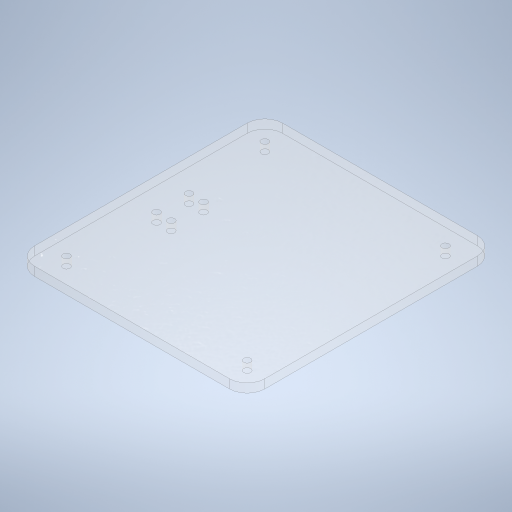
# Autodesk Inventor part: base
Saved by Autodesk Inventor 2023.1 (Build 271208000, 208)
## iProperties
Created: 2023-05-03
Part Number: base
Material: Acrylic
Document SubType Name: Modeling
Designer: felip
Density: 1.188 g/cm^3
Appearance: Transparent - Clear
Author: felip
Autodesk Inventor part; units mm, degrees
ref_plane "YZ Plane" through (0, 0, 0) normal (1, 0, 0) x (0, 1, 0)
ref_plane "XZ Plane" through (0, 0, 0) normal (0, 1, 0) x (-1, 0, 0)
ref_plane "XY Plane" through (0, 0, 0) normal (0, 0, 1) x (1, 0, 0)
sketch "Sketch1" plane through (0, 0, 0) normal (0, 1, 0) x (-1, 0, 0)
  line L0 (65, 70) -> (-65, 70)
  line L1 (-65, 70) -> (-65, -70)
  line L2 (-65, -70) -> (65, -70)
  line L3 (65, -70) -> (65, 70)
  circle A0 centre (51, 56) radius 2
  line L4 (0, 0) -> (22.2667, 0) construction
  line L5 (0, 25.5634) -> (0, -25.157) construction
  circle A1 centre (51, -56) radius 2
  circle A2 centre (-51, 56) radius 2
  circle A3 centre (-51, -56) radius 2
  circle A4 centre (47, 9.15) radius 2
  circle A5 centre (38.75, 9.15) radius 2
  circle A6 centre (47, -9.15) radius 2
  circle A7 centre (38.75, -9.15) radius 2
  dimension "d0" = 140
  dimension "d1" = 130
  dimension "d2" = 4
  dimension "d3" = 14
  dimension "d4" = 14
  dimension "d5" = 70
  dimension "d6" = 65
  dimension "d9" = 18
  dimension "d10" = 4
  dimension "d11" = 9.15
  dimension "d12" = 4
  dimension "d13" = 9.15
  dimension "d14" = 8.25
  constraints: 12 end point, 8 centre point, 5 symmetric about line, 2 horizontal, 2 parallel, 1 perpendicular, 1 vertical, 5 other
  measures "d0" distance of L0.end L1.end
  measures "d1" distance of L0.start L0.end
  measures "d2" diameter of A0
  measures "d3" distance from line of L3 A0.centre
  measures "d4" distance from line of L0 A0.centre
  measures "d5" distance from line of L0 L4.start
  measures "d6" distance from line of L3 L4.start
  measures "d9" distance from line of A4.centre L3
  measures "d10" diameter of A4
  measures "d11" distance from line of A4.centre L4
  measures "d12" diameter of A5
  measures "d13" distance from line of L4 A5.centre
  measures "d14" distance of A4.centre A5.centre
extrude "Extrusion1" add sketch "Sketch1" along normal blind 5
fillet "Fillet1" radius 10 4 edges at (65, 2.5, 70) (65, 2.5, -70) (-65, 2.5, -70) (-65, 2.5, 70)
equation "\"d4\" = d3"
equation "\"d5\" = 0.5 * d0"
equation "\"d6\" = 0.5 * d1"
equation "\"d13\" = d11"
body "Solid1"
